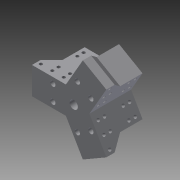
# Autodesk Inventor part: core2
Saved by Autodesk Inventor 2015 (Build 190159000, 159)
## iProperties
Created: 2015-10-17
Part Number: core2
Material: ABS Plastic
Document SubType Name: Modeling
Designer: Brian
Density: 1.06 g/cm^3
Appearance: Default
Mass: 80.6745 g
Surface Area: 258.66 cm^2
Volume: 76.108 cm^3
Author: Brian
Autodesk Inventor part; units mm, degrees
ref_plane "YZ Plane" through (0, 0, 0) normal (1, 0, 0) x (0, 1, 0)
ref_plane "XZ Plane" through (0, 0, 0) normal (0, 1, 0) x (-1, 0, 0)
ref_plane "XY Plane" through (0, 0, 0) normal (0, 0, 1) x (1, 0, 0)
sketch "Sketch1" plane through (0, 0, 0) normal (0, 1, 0) x (-1, 0, 0)
  line L0 (29.5056, 13) -> (7.5056, 13)
  line L1 (7.5056, 13) -> (7.5056, -13) construction
  line L2 (7.5056, -13) -> (29.5056, -13)
  line L3 (29.5056, -13) -> (29.5056, 13)
  line L4 (7.5056, 13) -> (-15.0111, 0) construction
  line L5 (-15.0111, 0) -> (-26.0111, 19.0526)
  line L6 (-26.0111, 19.0526) -> (-3.4944, 32.0526)
  line L7 (-3.4944, 32.0526) -> (7.5056, 13)
  line L8 (-15.0111, 0) -> (7.5056, -13) construction
  line L9 (7.5056, -13) -> (-3.4944, -32.0526)
  line L10 (-3.4944, -32.0526) -> (-26.0111, -19.0526)
  line L11 (-26.0111, -19.0526) -> (-15.0111, 0)
  line L12 (7.5056, 13) -> (-3.7528, -6.5) construction
  point P0 (0, 0)
  point P1 (29.5056, 0)
  dimension "d0" = 26
  dimension "d1" = 60
  dimension "d2" = 22
  dimension "d3" = 22
  dimension "d4" = 22
  constraints: 26 end point, 6 parallel, 3 perpendicular, 2 horizontal alignment, 2 midpoint, 1 horizontal, 1 point on line
  measures "d0" distance of L2.end L0.start
  measures "d1" angle of L1 L4
  measures "d2" distance of L1.end L2.end
  measures "d3" distance of L1.end L9.end
  measures "d4" distance of L4.end L5.end
extrude "Extrusion1" add sketch "Sketch1" along normal blind 40
sketch "Sketch2" plane through (-7.5056, 0, -13) normal (0, 0, -1) x (-1, 0, 0)
  line L0 (0, 0) -> (22, 0) projected
  line L1 (22, 0) -> (22, 40) projected
  line L2 (0, 40) -> (22, 40) projected
  line L3 (0, 0) -> (0, 40) projected
  line L4 (22, 0) -> (22, 40) projected
  line L5 (22, 18.5) -> (32.5, 8)
  line L6 (32.5, 0) -> (22, 0)
  line L7 (32.5, 8) -> (32.5, 0)
  line L8 (32.5, 8) -> (40.5, 0)
  point P0 (-7.5056, 0)
  dimension "d7" = 45
  dimension "d14" = 8
  dimension "d15" = 18.5
  constraints: 8 end point, 2 perpendicular, 2 point on line, 1 collinear
  measures "d7" angle of L6 L5
  measures "d14" distance of L5.end L6.start
  measures "d15" distance of L0.end L8.end
extrude "Extrusion2" add sketch "Sketch2" against normal up to surface (26 mm away)
pattern_circular "Circular Pattern1" count 3 over 360 about axis through (0, -10, 0) along (0, 1, 0) of "Extrusion2"
sketch "Sketch3" plane through (0, 40, 0) normal (0, 1, 0) x (1, 0, 0)
  circle A0 centre (0, 0) radius 4
  dimension "d17" = 8
  constraints: 1 centre point
  measures "d17" diameter of A0
extrude "Extrusion3" cut sketch "Sketch3" against normal blind 100
sketch "Sketch4" plane through (-7.5056, 40, -13) normal (0, 0, -1) x (-1, 0, 0)
  circle A0 centre (18, -5) radius 1.5
  line L0 (18, -5) -> (18, -35) construction
  line L1 (18, -35) -> (7, -35) construction
  line L2 (7, -35) -> (7, -5) construction
  line L3 (7, -5) -> (18, -5) construction
  circle A1 centre (7, -5) radius 1.5
  circle A2 centre (7, -35) radius 1.5
  circle A3 centre (18, -35) radius 1.5
  circle A4 centre (29, -35) radius 1.5
  circle A5 centre (7, -11) radius 1.5
  circle A6 centre (18, -11) radius 1.5
  circle A7 centre (7, -29) radius 1.5
  circle A8 centre (18, -29) radius 1.5
  line L4 (0, -40) -> (32.5, -40) projected
  line L5 (32.5, -40) -> (32.5, -32) projected
  line L6 (32.5, -32) -> (22, -21.5) projected
  line L7 (22, -21.5) -> (22, 0) projected
  line L8 (0, 0) -> (22, 0) projected
  line L9 (0, -40) -> (0, 0) projected
  point P0 (-7.5056, -40)
  dimension "d20" = 3
  dimension "d21" = 3
  dimension "d22" = 3
  dimension "d23" = 3
  dimension "d24" = 3
  dimension "d25" = 3
  dimension "d26" = 3
  dimension "d27" = 3
  dimension "d28" = 3
  dimension "d29" = 5
  dimension "d30" = 5
  dimension "d31" = 6
  dimension "d32" = 6
  dimension "d33" = 11
  dimension "d34" = 7
  dimension "d35" = 4
  constraints: 9 centre point, 8 end point, 4 point on line, 3 coincident, 3 horizontal alignment, 2 parallel, 1 perpendicular, 1 vertical
  measures "d20" diameter of A0
  measures "d21" diameter of A8
  measures "d22" diameter of A6
  measures "d23" diameter of A3
  measures "d24" diameter of A2
  measures "d25" diameter of A7
  measures "d26" diameter of A5
  measures "d27" diameter of A1
  measures "d28" diameter of A4
  measures "d29" distance between parallel lines of L8 L3
  measures "d30" distance between parallel lines of L4 L1
  measures "d31" distance of L2.end A5.centre
  measures "d32" distance of L1.end A7.centre
  measures "d33" distance of L0.end A4.centre
  measures "d34" distance between parallel lines of L9 L2
  measures "d35" distance between parallel lines of L7 L0
extrude "Extrusion4" cut sketch "Sketch4" against normal blind 100 contours A0 | A1 | A2 | A3 | A4 | A5 | A6 | A7 | A8
sketch "Sketch5" plane through (0, 40, 0) normal (0, 1, 0) x (1, 0, 0)
  circle A0 centre (0, 0) radius 4 projected
  line L0 (15.0111, 0) -> (26.0111, 19.0526) projected
  line L1 (26.0111, 19.0526) -> (3.4944, 32.0526) projected
  line L2 (3.4944, 32.0526) -> (-7.5056, 13) projected
  line L3 (-7.5056, 13) -> (-29.5056, 13) projected
  line L4 (-29.5056, 13) -> (-29.5056, -13) projected
  line L5 (-29.5056, -13) -> (-7.5056, -13) projected
  line L6 (-7.5056, -13) -> (3.4944, -32.0526) projected
  line L7 (3.4944, -32.0526) -> (26.0111, -19.0526) projected
  line L8 (26.0111, -19.0526) -> (15.0111, 0) projected
  circle A1 centre (-20.0056, -7.5) radius 2.5
  circle A2 centre (-20.0056, 7.5) radius 2.5
  dimension "d38" = 5
  dimension "d39" = 5
  dimension "d40" = 5.5
  dimension "d41" = 5.5
  dimension "d42" = 9.5
  constraints: 2 centre point, 1 vertical alignment
  measures "d38" diameter of A1
  measures "d39" diameter of A2
  measures "d40" distance from line of L5 A1.centre
  measures "d41" distance from line of L3 A2.centre
  measures "d42" distance from line of L4 A2.centre
extrude "Extrusion5" cut sketch "Sketch5" against normal blind 100 contours A1 | A2
pattern_circular "Circular Pattern2" count 3 over 360 about axis through (0, -10, 0) along (0, 1, 0) of "Extrusion5"
sketch "Sketch6" plane through (0, 40, 0) normal (0, 1, 0) x (1, 0, 0)
  line L0 (6.4, -6.4) -> (6.4, 6.4)
  line L1 (6.4, 6.4) -> (-6.4, 6.4)
  line L2 (-6.4, 6.4) -> (-6.4, -6.4)
  line L3 (-6.4, -6.4) -> (6.4, -6.4)
  line L4 (6.4, -6.4) -> (-6.4, 6.4) construction
  point P0 (0, 0)
  point P1 (0, 0)
  dimension "d48" = 12.8
  dimension "d49" = 12.8
  constraints: 10 end point, 2 parallel, 1 coincident, 1 midpoint, 1 perpendicular, 1 vertical
  measures "d48" distance of L0.end L1.end
  measures "d49" distance of L0.start L0.end
extrude "Extrusion6" cut sketch "Sketch6" against normal blind 30
pattern_circular "Circular Pattern3" count 3 over 360 about axis through (0, -10, 0) along (0, 1, 0) of "Extrusion4"
equation "\"d3\" = d2"
equation "\"d4\" = d2"
equation "\"d21\" = d20"
equation "\"d22\" = d20"
equation "\"d23\" = d20"
equation "\"d24\" = d20"
equation "\"d25\" = d20"
equation "\"d26\" = d20"
equation "\"d27\" = d20"
equation "\"d28\" = d20"
equation "\"d39\" = d38"
equation "\"d41\" = d40"
equation "\"d49\" = d48"
body "Solid1"
